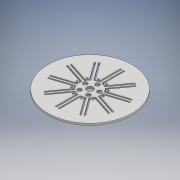
# Autodesk Inventor part: Torque Spring
Saved by Autodesk Inventor 2017 (Build 210142000, 142)
## iProperties
Created: 2019-11-16
Part Number: Torque Spring
Material: Generic
Document SubType Name: Modeling
Designer: Dell
Density: 1 g/cm^3
Appearance: Default
Author: Dell
Autodesk Inventor part; units mm, degrees
ref_plane "YZ Plane" through (0, 0, 0) normal (1, 0, 0) x (0, 1, 0)
ref_plane "XZ Plane" through (0, 0, 0) normal (0, 1, 0) x (-1, 0, 0)
ref_plane "XY Plane" through (0, 0, 0) normal (0, 0, 1) x (1, 0, 0)
sketch "Sketch1" plane through (0, 0, 0) normal (0, 0, 1) x (1, 0, 0)
  circle A0 centre (0, 0) radius 3.5
  circle A1 centre (0, 8) radius 2.25
  circle A2 centre (-7.6085, 2.4721) radius 2.25
  circle A3 centre (-4.7023, -6.4721) radius 2.25
  circle A4 centre (4.7023, -6.4721) radius 2.25
  circle A5 centre (7.6085, 2.4721) radius 2.25
  circle A6 centre (0, 0) radius 11.5 construction
  circle A7 centre (0, 0) radius 25
  circle A8 centre (0, 0) radius 20 construction
  circle A9 centre (14, 0) radius 1
  circle A10 centre (14, 0) radius 2
  line L0 (14, 2) -> (19.8997, 2)
  line L1 (14, -2) -> (19.8997, -2)
  arc A11 (19.8997, -2) -> (19.8997, 2) centre (0, 0) ccw construction
  circle A12 centre (11.3262, 8.229) radius 1
  circle A13 centre (11.3262, 8.229) radius 2
  line L2 (10.1507, 9.847) -> (14.9237, 13.3148)
  arc A14 (17.2748, 10.0787) -> (14.9237, 13.3148) centre (0, 0) ccw construction
  line L3 (12.5018, 6.611) -> (17.2748, 10.0787)
  circle A15 centre (4.3262, 13.3148) radius 1
  circle A16 centre (4.3262, 13.3148) radius 2
  line L4 (2.4241, 13.9328) -> (4.2472, 19.5438)
  arc A17 (8.0515, 18.3078) -> (4.2472, 19.5438) centre (0, 0) ccw
  line L5 (6.2284, 12.6968) -> (8.0515, 18.3078)
  circle A18 centre (-4.3262, 13.3148) radius 1
  circle A19 centre (-4.3262, 13.3148) radius 2
  line L6 (-6.2284, 12.6968) -> (-8.0515, 18.3078)
  arc A20 (-4.2472, 19.5438) -> (-8.0515, 18.3078) centre (0, 0) ccw
  line L7 (-2.4241, 13.9328) -> (-4.2472, 19.5438)
  circle A21 centre (-11.3262, 8.229) radius 1
  circle A22 centre (-11.3262, 8.229) radius 2
  line L8 (-12.5018, 6.611) -> (-17.2748, 10.0787)
  arc A23 (-14.9237, 13.3148) -> (-17.2748, 10.0787) centre (0, 0) ccw
  line L9 (-10.1507, 9.847) -> (-14.9237, 13.3148)
  circle A24 centre (-14, 0) radius 1
  circle A25 centre (-14, 0) radius 2
  line L10 (-14, -2) -> (-19.8997, -2)
  arc A26 (-19.8997, 2) -> (-19.8997, -2) centre (0, 0) ccw
  line L11 (-14, 2) -> (-19.8997, 2)
  circle A27 centre (-11.3262, -8.229) radius 1
  circle A28 centre (-11.3262, -8.229) radius 2
  line L12 (-10.1507, -9.847) -> (-14.9237, -13.3148)
  arc A29 (-17.2748, -10.0787) -> (-14.9237, -13.3148) centre (0, 0) ccw
  line L13 (-12.5018, -6.611) -> (-17.2748, -10.0787)
  circle A30 centre (-4.3262, -13.3148) radius 1
  circle A31 centre (-4.3262, -13.3148) radius 2
  line L14 (-2.4241, -13.9328) -> (-4.2472, -19.5438)
  arc A32 (-8.0515, -18.3078) -> (-4.2472, -19.5438) centre (0, 0) ccw
  line L15 (-6.2284, -12.6968) -> (-8.0515, -18.3078)
  circle A33 centre (4.3262, -13.3148) radius 1
  circle A34 centre (4.3262, -13.3148) radius 2
  line L16 (6.2284, -12.6968) -> (8.0515, -18.3078)
  arc A35 (4.2472, -19.5438) -> (8.0515, -18.3078) centre (0, 0) ccw
  line L17 (2.4241, -13.9328) -> (4.2472, -19.5438)
  circle A36 centre (11.3262, -8.229) radius 1
  circle A37 centre (11.3262, -8.229) radius 2
  line L18 (12.5018, -6.611) -> (17.2748, -10.0787)
  arc A38 (14.9237, -13.3148) -> (17.2748, -10.0787) centre (0, 0) ccw
  line L19 (10.1507, -9.847) -> (14.9237, -13.3148)
  line L20 (-0.75, 11.4755) -> (-0.75, 19.9859)
  line L21 (0.75, 19.9859) -> (0.75, 11.4755)
  line L22 (-0.75, 19.9859) -> (0.75, 19.9859) construction
  arc A39 (-0.75, 19.9859) -> (-4.2472, 19.5438) centre (0, 0) ccw
  arc A40 (4.2472, 19.5438) -> (0.75, 19.9859) centre (0, 0) ccw
  arc A41 (-8.0515, 18.3078) -> (-11.1407, 16.6098) centre (0, 0) ccw
  line L23 (-12.3542, 15.7281) -> (-11.1407, 16.6098) construction
  arc A42 (-12.3542, 15.7281) -> (-14.9237, 13.3148) centre (0, 0) ccw
  line L24 (-7.3519, 8.843) -> (-12.3542, 15.7281)
  line L25 (-11.1407, 16.6098) -> (-6.1384, 9.7247)
  arc A43 (-17.2748, 10.0787) -> (-18.776, 6.8893) centre (0, 0) ccw
  line L26 (-19.2395, 5.4627) -> (-18.776, 6.8893) construction
  arc A44 (-19.2395, 5.4627) -> (-19.8997, 2) centre (0, 0) ccw
  line L27 (-11.1456, 2.8328) -> (-19.2395, 5.4627)
  line L28 (-18.776, 6.8893) -> (-10.6821, 4.2594)
  arc A45 (-19.8997, -2) -> (-19.2395, -5.4627) centre (0, 0) ccw
  line L29 (-18.776, -6.8893) -> (-19.2395, -5.4627) construction
  arc A46 (-18.776, -6.8893) -> (-17.2748, -10.0787) centre (0, 0) ccw
  line L30 (-10.6821, -4.2594) -> (-18.776, -6.8893)
  line L31 (-19.2395, -5.4627) -> (-11.1456, -2.8328)
  arc A47 (-14.9237, -13.3148) -> (-12.3542, -15.7281) centre (0, 0) ccw
  line L32 (-11.1407, -16.6098) -> (-12.3542, -15.7281) construction
  arc A48 (-11.1407, -16.6098) -> (-8.0515, -18.3078) centre (0, 0) ccw
  line L33 (-6.1384, -9.7247) -> (-11.1407, -16.6098)
  line L34 (-12.3542, -15.7281) -> (-7.3519, -8.843)
  arc A49 (-4.2472, -19.5438) -> (-0.75, -19.9859) centre (0, 0) ccw
  line L35 (0.75, -19.9859) -> (-0.75, -19.9859) construction
  arc A50 (0.75, -19.9859) -> (4.2472, -19.5438) centre (0, 0) ccw
  line L36 (0.75, -11.4755) -> (0.75, -19.9859)
  line L37 (-0.75, -19.9859) -> (-0.75, -11.4755)
  arc A51 (8.0515, -18.3078) -> (11.1407, -16.6098) centre (0, 0) ccw
  line L38 (12.3542, -15.7281) -> (11.1407, -16.6098) construction
  arc A52 (12.3542, -15.7281) -> (14.9237, -13.3148) centre (0, 0) ccw
  line L39 (7.3519, -8.843) -> (12.3542, -15.7281)
  line L40 (11.1407, -16.6098) -> (6.1384, -9.7247)
  arc A53 (17.2748, -10.0787) -> (18.776, -6.8893) centre (0, 0) ccw
  line L41 (19.2395, -5.4627) -> (18.776, -6.8893) construction
  arc A54 (19.2395, -5.4627) -> (19.8997, -2) centre (0, 0) ccw
  line L42 (11.1456, -2.8328) -> (19.2395, -5.4627)
  line L43 (18.776, -6.8893) -> (10.6821, -4.2594)
  arc A55 (19.8997, 2) -> (19.2395, 5.4627) centre (0, 0) ccw
  line L44 (18.776, 6.8893) -> (19.2395, 5.4627) construction
  arc A56 (18.776, 6.8893) -> (17.2748, 10.0787) centre (0, 0) ccw
  line L45 (10.6821, 4.2594) -> (18.776, 6.8893)
  line L46 (19.2395, 5.4627) -> (11.1456, 2.8328)
  arc A57 (14.9237, 13.3148) -> (12.3542, 15.7281) centre (0, 0) ccw
  line L47 (11.1407, 16.6098) -> (12.3542, 15.7281) construction
  arc A58 (11.1407, 16.6098) -> (8.0515, 18.3078) centre (0, 0) ccw
  line L48 (6.1384, 9.7247) -> (11.1407, 16.6098)
  line L49 (12.3542, 15.7281) -> (7.3519, 8.843)
  arc A59 (6.1384, 9.7247) -> (0.75, 11.4755) centre (0, 0) ccw
  circle A60 centre (0, 0) radius 11.5 construction
  arc A61 (-0.75, 11.4755) -> (-6.1384, 9.7247) centre (0, 0) ccw
  circle A62 centre (0, 0) radius 11.5 construction
  arc A63 (-7.3519, 8.843) -> (-10.6821, 4.2594) centre (0, 0) ccw
  circle A64 centre (0, 0) radius 11.5 construction
  arc A65 (-11.1456, 2.8328) -> (-11.1456, -2.8328) centre (0, 0) ccw
  circle A66 centre (0, 0) radius 11.5 construction
  arc A67 (-10.6821, -4.2594) -> (-7.3519, -8.843) centre (0, 0) ccw
  circle A68 centre (0, 0) radius 11.5 construction
  arc A69 (-6.1384, -9.7247) -> (-0.75, -11.4755) centre (0, 0) ccw
  circle A70 centre (0, 0) radius 11.5 construction
  arc A71 (0.75, -11.4755) -> (6.1384, -9.7247) centre (0, 0) ccw
  circle A72 centre (0, 0) radius 11.5 construction
  arc A73 (7.3519, -8.843) -> (10.6821, -4.2594) centre (0, 0) ccw
  circle A74 centre (0, 0) radius 11.5 construction
  arc A75 (11.1456, -2.8328) -> (11.1456, 2.8328) centre (0, 0) ccw
  circle A76 centre (0, 0) radius 11.5 construction
  arc A77 (10.6821, 4.2594) -> (7.3519, 8.843) centre (0, 0) ccw
  point P0 (0, 19.9859)
  point P1 (-11.7474, 16.169)
  point P2 (-19.0078, 6.176)
  point P3 (-19.0078, -6.176)
  point P4 (-11.7474, -16.169)
  point P5 (0, -19.9859)
  point P6 (11.7474, -16.169)
  point P7 (19.0078, -6.176)
  point P8 (19.0078, 6.176)
  point P9 (11.7474, 16.169)
  dimension "d0" = 7
  dimension "d1" = 4.5
  dimension "d2" = 8
  dimension "d5" = 360
  dimension "d7" = 23
  dimension "d8" = 50
  dimension "d9" = 40
  dimension "d10" = 2
  dimension "d11" = 14
  dimension "d12" = 4
  dimension "d15" = 360
  dimension "d17" = 1.5
  dimension "d20" = 360
  dimension "d24" = 360
  constraints: 134 point on circle, 100 end point, 78 centre point, 17 coincident, 2 midpoint, 2 parallel, 2 tangent, 2 vertical alignment, 1 concentric, 1 horizontal, 1 horizontal alignment, 1 perpendicular, 1 point on line, 1 vertical, 344 other
  measures "d0" diameter of A0
  measures "d1" diameter of A1
  measures "d2" distance of point (0, 0) A1.centre
  measures "d7" diameter of A6
  measures "d8" diameter of A7
  measures "d9" diameter of A8
  measures "d10" diameter of A9
  measures "d11" distance of point (0, 0) A9.centre
  measures "d12" diameter of A10
  measures "d17" distance between parallel lines of L21 L20
sketch "Sketch2" plane through (0, 0, 0) normal (0, 0, 1) x (1, 0, 0)
  circle A0 centre (0, 0) radius 3.5
  circle A1 centre (0, 8) radius 2.25
  circle A2 centre (14, 0) radius 2 construction
  line L0 (13.382, 1.9021) -> (33.9322, 8.5793)
  line L1 (13.382, -1.9021) -> (33.9322, -8.5793)
  line L2 (11.2047, 2.5892) -> (33.5824, 9.8601)
  line L3 (11.2047, -2.5892) -> (33.5824, -9.8601)
  arc A3 (11.2047, -2.5892) -> (11.2047, 2.5892) centre (0, 0) ccw
  arc A4 (33.5824, -9.8601) -> (33.5824, 9.8601) centre (0, 0) ccw construction
  arc A5 (33.9322, 8.5793) -> (33.5824, 9.8601) centre (0, 0) ccw
  arc A6 (33.5824, -9.8601) -> (33.9322, -8.5793) centre (0, 0) ccw
  circle A7 centre (-7.6085, 2.4721) radius 2.25
  circle A8 centre (-4.7023, -6.4721) radius 2.25
  circle A9 centre (4.7023, -6.4721) radius 2.25
  circle A10 centre (7.6085, 2.4721) radius 2.25
  arc A11 (13.382, 1.9021) -> (13.382, -1.9021) centre (14, 0) ccw
  circle A12 centre (14, 0) radius 1
  circle A13 centre (0, 0) radius 45
  arc A14 (10.5867, 4.4913) -> (7.5429, 8.6807) centre (0, 0) ccw
  line L4 (7.5429, 8.6807) -> (21.3731, 27.7162)
  line L5 (9.7082, 9.4046) -> (22.409, 26.8857)
  arc A15 (22.409, 26.8857) -> (21.3731, 27.7162) centre (0, 0) ccw
  arc A16 (32.9644, 11.7622) -> (21.3731, 27.7162) centre (0, 0) ccw construction
  line L6 (11.9443, 6.3269) -> (32.4945, 13.0041)
  arc A17 (32.9644, 11.7622) -> (32.4945, 13.0041) centre (0, 0) ccw
  line L7 (10.5867, 4.4913) -> (32.9644, 11.7622)
  arc A18 (9.7082, 9.4046) -> (11.9443, 6.3269) centre (11.3262, 8.229) ccw
  circle A19 centre (11.3262, 8.229) radius 1
  circle A20 centre (11.3262, 8.229) radius 2 construction
  arc A21 (5.9249, 9.8562) -> (1, 11.4564) centre (0, 0) ccw
  line L8 (1, 11.4564) -> (1, 34.9857)
  line L9 (2.3262, 13.3148) -> (2.3262, 34.9226)
  arc A22 (2.3262, 34.9226) -> (1, 34.9857) centre (0, 0) ccw
  arc A23 (19.7551, 28.8918) -> (1, 34.9857) centre (0, 0) ccw construction
  line L10 (5.9443, 12.1392) -> (18.645, 29.6203)
  arc A24 (19.7551, 28.8918) -> (18.645, 29.6203) centre (0, 0) ccw
  line L11 (5.9249, 9.8562) -> (19.7551, 28.8918)
  arc A25 (2.3262, 13.3148) -> (5.9443, 12.1392) centre (4.3262, 13.3148) ccw
  circle A26 centre (4.3262, 13.3148) radius 1
  circle A27 centre (4.3262, 13.3148) radius 2 construction
  arc A28 (-1, 11.4564) -> (-5.9249, 9.8562) centre (0, 0) ccw
  line L12 (-5.9249, 9.8562) -> (-19.7551, 28.8918)
  line L13 (-5.9443, 12.1392) -> (-18.645, 29.6203)
  arc A29 (-18.645, 29.6203) -> (-19.7551, 28.8918) centre (0, 0) ccw
  arc A30 (-1, 34.9857) -> (-19.7551, 28.8918) centre (0, 0) ccw construction
  line L14 (-2.3262, 13.3148) -> (-2.3262, 34.9226)
  arc A31 (-1, 34.9857) -> (-2.3262, 34.9226) centre (0, 0) ccw
  line L15 (-1, 11.4564) -> (-1, 34.9857)
  arc A32 (-5.9443, 12.1392) -> (-2.3262, 13.3148) centre (-4.3262, 13.3148) ccw
  circle A33 centre (-4.3262, 13.3148) radius 1
  circle A34 centre (-4.3262, 13.3148) radius 2 construction
  arc A35 (-7.5429, 8.6807) -> (-10.5867, 4.4913) centre (0, 0) ccw
  line L16 (-10.5867, 4.4913) -> (-32.9644, 11.7622)
  line L17 (-11.9443, 6.3269) -> (-32.4945, 13.0041)
  arc A36 (-32.4945, 13.0041) -> (-32.9644, 11.7622) centre (0, 0) ccw
  arc A37 (-21.3731, 27.7162) -> (-32.9644, 11.7622) centre (0, 0) ccw construction
  line L18 (-9.7082, 9.4046) -> (-22.409, 26.8857)
  arc A38 (-21.3731, 27.7162) -> (-22.409, 26.8857) centre (0, 0) ccw
  line L19 (-7.5429, 8.6807) -> (-21.3731, 27.7162)
  arc A39 (-11.9443, 6.3269) -> (-9.7082, 9.4046) centre (-11.3262, 8.229) ccw
  circle A40 centre (-11.3262, 8.229) radius 1
  circle A41 centre (-11.3262, 8.229) radius 2 construction
  arc A42 (-11.2047, 2.5892) -> (-11.2047, -2.5892) centre (0, 0) ccw
  line L20 (-11.2047, -2.5892) -> (-33.5824, -9.8601)
  line L21 (-13.382, -1.9021) -> (-33.9322, -8.5793)
  arc A43 (-33.9322, -8.5793) -> (-33.5824, -9.8601) centre (0, 0) ccw
  arc A44 (-33.5824, 9.8601) -> (-33.5824, -9.8601) centre (0, 0) ccw construction
  line L22 (-13.382, 1.9021) -> (-33.9322, 8.5793)
  arc A45 (-33.5824, 9.8601) -> (-33.9322, 8.5793) centre (0, 0) ccw
  line L23 (-11.2047, 2.5892) -> (-33.5824, 9.8601)
  arc A46 (-13.382, -1.9021) -> (-13.382, 1.9021) centre (-14, 0) ccw
  circle A47 centre (-14, 0) radius 1
  circle A48 centre (-14, 0) radius 2 construction
  arc A49 (-10.5867, -4.4913) -> (-7.5429, -8.6807) centre (0, 0) ccw
  line L24 (-7.5429, -8.6807) -> (-21.3731, -27.7162)
  line L25 (-9.7082, -9.4046) -> (-22.409, -26.8857)
  arc A50 (-22.409, -26.8857) -> (-21.3731, -27.7162) centre (0, 0) ccw
  arc A51 (-32.9644, -11.7622) -> (-21.3731, -27.7162) centre (0, 0) ccw construction
  line L26 (-11.9443, -6.3269) -> (-32.4945, -13.0041)
  arc A52 (-32.9644, -11.7622) -> (-32.4945, -13.0041) centre (0, 0) ccw
  line L27 (-10.5867, -4.4913) -> (-32.9644, -11.7622)
  arc A53 (-9.7082, -9.4046) -> (-11.9443, -6.3269) centre (-11.3262, -8.229) ccw
  circle A54 centre (-11.3262, -8.229) radius 1
  circle A55 centre (-11.3262, -8.229) radius 2 construction
  arc A56 (-5.9249, -9.8562) -> (-1, -11.4564) centre (0, 0) ccw
  line L28 (-1, -11.4564) -> (-1, -34.9857)
  line L29 (-2.3262, -13.3148) -> (-2.3262, -34.9226)
  arc A57 (-2.3262, -34.9226) -> (-1, -34.9857) centre (0, 0) ccw
  arc A58 (-19.7551, -28.8918) -> (-1, -34.9857) centre (0, 0) ccw construction
  line L30 (-5.9443, -12.1392) -> (-18.645, -29.6203)
  arc A59 (-19.7551, -28.8918) -> (-18.645, -29.6203) centre (0, 0) ccw
  line L31 (-5.9249, -9.8562) -> (-19.7551, -28.8918)
  arc A60 (-2.3262, -13.3148) -> (-5.9443, -12.1392) centre (-4.3262, -13.3148) ccw
  circle A61 centre (-4.3262, -13.3148) radius 1
  circle A62 centre (-4.3262, -13.3148) radius 2 construction
  arc A63 (1, -11.4564) -> (5.9249, -9.8562) centre (0, 0) ccw
  line L32 (5.9249, -9.8562) -> (19.7551, -28.8918)
  line L33 (5.9443, -12.1392) -> (18.645, -29.6203)
  arc A64 (18.645, -29.6203) -> (19.7551, -28.8918) centre (0, 0) ccw
  arc A65 (1, -34.9857) -> (19.7551, -28.8918) centre (0, 0) ccw construction
  line L34 (2.3262, -13.3148) -> (2.3262, -34.9226)
  arc A66 (1, -34.9857) -> (2.3262, -34.9226) centre (0, 0) ccw
  line L35 (1, -11.4564) -> (1, -34.9857)
  arc A67 (5.9443, -12.1392) -> (2.3262, -13.3148) centre (4.3262, -13.3148) ccw
  circle A68 centre (4.3262, -13.3148) radius 1
  circle A69 centre (4.3262, -13.3148) radius 2 construction
  arc A70 (7.5429, -8.6807) -> (10.5867, -4.4913) centre (0, 0) ccw
  line L36 (10.5867, -4.4913) -> (32.9644, -11.7622)
  line L37 (11.9443, -6.3269) -> (32.4945, -13.0041)
  arc A71 (32.4945, -13.0041) -> (32.9644, -11.7622) centre (0, 0) ccw
  arc A72 (21.3731, -27.7162) -> (32.9644, -11.7622) centre (0, 0) ccw construction
  line L38 (9.7082, -9.4046) -> (22.409, -26.8857)
  arc A73 (21.3731, -27.7162) -> (22.409, -26.8857) centre (0, 0) ccw
  line L39 (7.5429, -8.6807) -> (21.3731, -27.7162)
  arc A74 (11.9443, -6.3269) -> (9.7082, -9.4046) centre (11.3262, -8.229) ccw
  circle A75 centre (11.3262, -8.229) radius 1
  circle A76 centre (11.3262, -8.229) radius 2 construction
  point P0 (11.5, 0)
  point P1 (35, 0)
  point P2 (9.3037, 6.7595)
  point P3 (28.3156, 20.5725)
  point P4 (3.5537, 10.9371)
  point P5 (10.8156, 33.287)
  point P6 (-3.5537, 10.9371)
  point P7 (-10.8156, 33.287)
  point P8 (-9.3037, 6.7595)
  point P9 (-28.3156, 20.5725)
  point P10 (-11.5, 0)
  point P11 (-35, 0)
  point P12 (-9.3037, -6.7595)
  point P13 (-28.3156, -20.5725)
  point P14 (-3.5537, -10.9371)
  point P15 (-10.8156, -33.287)
  point P16 (3.5537, -10.9371)
  point P17 (10.8156, -33.287)
  point P18 (9.3037, -6.7595)
  point P19 (28.3156, -20.5725)
  dimension "d26" = 7
  dimension "d27" = 4.5
  dimension "d28" = 8
  dimension "d29" = 4
  dimension "d30" = 14
  dimension "d31" = 11.5
  dimension "d33" = 35
  dimension "d37" = 360
  dimension "d39" = 2
  dimension "d40" = 90
  dimension "d43" = 360
  dimension "d47" = 2
  dimension "d48" = 2
  constraints: 122 point on circle, 80 end point, 77 centre point, 16 coincident, 3 horizontal alignment, 3 tangent, 2 parallel, 1 vertical alignment, 292 other
  measures "d26" diameter of A0
  measures "d27" diameter of A1
  measures "d28" distance of point (0, 0) A1.centre
  measures "d29" diameter of A2
  measures "d30" distance of A2.centre point (0, 0)
  measures "d31" radius of A3
  measures "d33" radius of A4
  measures "d39" diameter of A12
  measures "d40" diameter of A13
  measures "d47" distance of L2.end L7.end
  measures "d48" distance of L2.start L7.start
extrude "Extrusion1" add sketch "Sketch2" along normal blind 2
body "Solid1"
